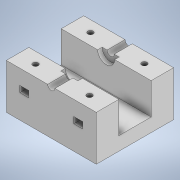
# Autodesk Inventor part: 19_Base_Pezzo_Unico
Saved by Autodesk Inventor 2020 (Build 240168000, 168)
## iProperties
Created: 2019-10-24
Part Number: 19_Base_Pezzo_Unico
Material: Generico
Document SubType Name: Modeling
Designer: socci
Density: 1 g/cm^3
Appearance: Default
Author: socci
Autodesk Inventor part; units mm, degrees
ref_plane "YZ Plane" through (0, 0, 0) normal (1, 0, 0) x (0, 1, 0)
ref_plane "XZ Plane" through (0, 0, 0) normal (0, 1, 0) x (-1, 0, 0)
ref_plane "XY Plane" through (0, 0, 0) normal (0, 0, 1) x (1, 0, 0)
sketch "Schizzo1" plane through (0, 0, 0) normal (0, 1, 0) x (-1, 0, 0)
  line L0 (50, 43) -> (-50, 43)
  line L1 (-50, 43) -> (-50, -43)
  line L2 (-50, -43) -> (50, -43)
  line L3 (50, -43) -> (50, 43)
  line L4 (50, 43) -> (-50, -43) construction
  line L5 (-50, 43) -> (50, -43) construction
  point P0 (0, 0)
  point P1 (0, 0)
  point P2 (0, 0)
  dimension "d0" = 100
  dimension "d1" = 86
  constraints: 12 end point, 3 midpoint, 2 parallel, 1 coincident, 1 horizontal, 1 perpendicular
  measures "d0" distance of L0.start L0.end
  measures "d1" distance of L2.end L0.start
extrude "Estrusione1" add sketch "Schizzo1" along normal blind 50
sketch "Schizzo2" plane through (50, 0, 43) normal (1, 0, 0) x (0, 0, -1)
  line L0 (43, 0) -> (43, 15)
  line L1 (25, 50) -> (61, 50)
  line L2 (61, 50) -> (61, 15)
  line L3 (61, 15) -> (25, 15)
  line L4 (25, 15) -> (25, 50)
  line L5 (25, 50) -> (61, 15) construction
  line L6 (61, 50) -> (25, 15) construction
  point P0 (43, 32.5)
  dimension "d4" = 15
  dimension "d5" = 36
  dimension "d6" = 35
  constraints: 14 end point, 3 midpoint, 2 parallel, 1 horizontal, 1 perpendicular, 1 vertical
  measures "d4" distance of L0.end L0.start
  measures "d5" distance of L1.start L1.end
  measures "d6" distance of L3.end L1.start
extrude "Estrusione2" cut sketch "Schizzo2" against normal blind 100
sketch "Schizzo3" plane through (50, 15, -18) normal (0, 0, 1) x (1, 0, 0)
  circle A0 centre (-50, 35) radius 9.5
  line L0 (0, 35) -> (-100, 35) projected
  point P0 (-50, -15)
  dimension "d9" = 19
  constraints: 1 centre point, 1 coincident, 1 midpoint
  measures "d9" diameter of A0
extrude "Estrusione3" cut sketch "Schizzo3" against normal blind 5
sketch "Schizzo4" plane through (50, 15, -23) normal (0, 0, 1) x (1, 0, 0)
  circle A0 centre (-50, 35) radius 4
  line L0 (0, 35) -> (-100, 35) projected
  point P0 (-50, -15)
  dimension "d12" = 8
  constraints: 1 centre point, 1 coincident, 1 midpoint
  measures "d12" diameter of A0
extrude "Estrusione4" cut sketch "Schizzo4" against normal blind 20
sketch "Schizzo5" plane through (50, 15, 18) normal (0, 0, -1) x (-1, 0, 0)
  circle A0 centre (50, 35) radius 9.5
  line L0 (100, 35) -> (0, 35) projected
  point P0 (50, -15)
  point P1 (50, 35)
  dimension "d15" = 19
  constraints: 1 centre point, 1 coincident, 1 midpoint
  measures "d15" diameter of A0
extrude "Estrusione5" cut sketch "Schizzo5" against normal blind 5
sketch "Schizzo6" plane through (50, 15, 23) normal (0, 0, -1) x (-1, 0, 0)
  circle A0 centre (50, 35) radius 4
  line L0 (40.5, 35) -> (59.5, 35) projected
  point P0 (50, -15)
  constraints: 1 centre point, 1 coincident, 1 midpoint
extrude "Estrusione6" cut sketch "Schizzo6" against normal blind 20
sketch "Schizzo7" plane through (0, 50, 0) normal (0, 1, 0) x (1, 0, 0)
  line L0 (-4, 43) -> (4, 43) projected
  line L1 (0, 43) -> (0, 18)
  line L2 (50, 18) -> (-50, 18) projected
  line L3 (-9.5, -18) -> (9.5, -18) projected
  line L4 (0, -18) -> (0, -43)
  line L5 (4, -43) -> (-4, -43) projected
  line L6 (-133, 18) -> (-97, 18) construction
  line L7 (-30, 30.5) -> (30, 30.5)
  line L8 (-30, -30.5) -> (30, -30.5)
  point P0 (0, 0)
  point P1 (0, 30.5)
  point P2 (0, -30.5)
  dimension "d22" = 60
  dimension "d23" = 60
  constraints: 10 end point, 8 midpoint, 2 perpendicular, 1 horizontal
  measures "d22" distance of L7.start L7.end
  measures "d23" distance of L8.start L8.end
hole "Foro1" at (-30, 50, -30.5) at (-30, 50, 30.5) at (30, 50, 30.5) at (30, 50, -30.5) direction (0, -1, 0) diameter 5.9 depth 35 tip angle 118 clearance for "Vite a testa esagonale" size "M5" standard "ANSI - Profilo M Metrico"
sketch "Schizzo8" plane through (-50, 0, 43) normal (0, 0, 1) x (1, 0, 0)
  line L0 (17.05, 50) -> (22.95, 50) projected
  line L1 (77.05, 50) -> (82.95, 50) projected
  line L2 (80, 50) -> (80, 30)
  line L3 (80, 50) -> (60, 50) construction
  line L4 (20, 50) -> (20, 30)
  line L5 (20, 50) -> (0, 50) construction
  line L6 (15, 33.5) -> (25, 33.5)
  line L7 (25, 33.5) -> (25, 26.5)
  line L8 (25, 26.5) -> (15, 26.5)
  line L9 (15, 26.5) -> (15, 33.5)
  line L10 (15, 33.5) -> (25, 26.5) construction
  line L11 (25, 33.5) -> (15, 26.5) construction
  line L12 (75, 33.5) -> (85, 33.5)
  line L13 (85, 33.5) -> (85, 26.5)
  line L14 (85, 26.5) -> (75, 26.5)
  line L15 (75, 26.5) -> (75, 33.5)
  line L16 (75, 33.5) -> (85, 26.5) construction
  line L17 (85, 33.5) -> (75, 26.5) construction
  point P0 (50, 0)
  point P1 (20, 30)
  dimension "d31" = 90
  dimension "d32" = 270
  dimension "d33" = 20
  dimension "d34" = 20
  dimension "d35" = 7
  dimension "d36" = 7
  dimension "d37" = 10
  dimension "d38" = 10
  constraints: 32 end point, 8 midpoint, 4 horizontal, 4 parallel, 4 perpendicular
  measures "d31" angle of L2 L3
  measures "d33" distance of L4.end L4.start
  measures "d34" distance of L2.end L2.start
  measures "d35" distance of L8.end L6.start
  measures "d36" distance of L12.end L13.end
  measures "d37" distance of L7.end L8.end
  measures "d38" distance of L13.end L14.end
extrude "Estrusione7" cut sketch "Schizzo8" against normal blind 19
sketch "Schizzo10" plane through (50, 0, -43) normal (0, 0, -1) x (-1, 0, 0)
  line L0 (17.05, 50) -> (22.95, 50)
  line L1 (77.05, 50) -> (82.95, 50)
  line L2 (80, 50) -> (80, 30)
  line L3 (80, 50) -> (60, 50) construction
  line L4 (20, 50) -> (20, 30)
  line L5 (20, 50) -> (0, 50) construction
  line L6 (15, 33.5) -> (25, 33.5)
  line L7 (25, 33.5) -> (25, 26.5)
  line L8 (25, 26.5) -> (15, 26.5)
  line L9 (15, 26.5) -> (15, 33.5)
  line L10 (15, 33.5) -> (25, 26.5) construction
  line L11 (25, 33.5) -> (15, 26.5) construction
  line L12 (75, 33.5) -> (85, 33.5)
  line L13 (85, 33.5) -> (85, 26.5)
  line L14 (85, 26.5) -> (75, 26.5)
  line L15 (75, 26.5) -> (75, 33.5)
  line L16 (75, 33.5) -> (85, 26.5) construction
  line L17 (85, 33.5) -> (75, 26.5) construction
  point P0 (50, 0)
  point P1 (50, 0)
  point P2 (20, 30)
  dimension "d42" = 90
  dimension "d43" = 270
  dimension "d44" = 20
  dimension "d45" = 20
  dimension "d46" = 7
  dimension "d47" = 7
  dimension "d48" = 10
  dimension "d49" = 10
  constraints: 36 end point, 8 midpoint, 4 horizontal, 4 parallel, 4 perpendicular
  measures "d42" angle of L2 L3
  measures "d44" distance of L4.end L4.start
  measures "d45" distance of L2.end L2.start
  measures "d46" distance of L8.end L6.start
  measures "d47" distance of L12.end L13.end
  measures "d48" distance of L7.end L8.end
  measures "d49" distance of L13.end L14.end
extrude "Estrusione8" cut sketch "Schizzo10" against normal blind 19
